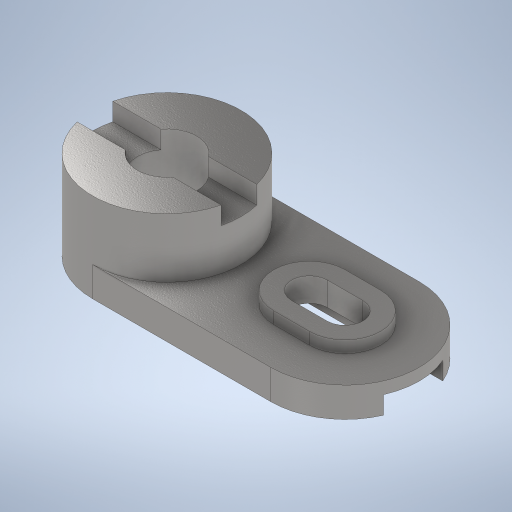
# Autodesk Inventor part: slider
Saved by Autodesk Inventor 2024 (Build 280153000, 153)
## iProperties
Created: 2024-02-08
Part Number: slider
Material: Stahl, galvanisiert
Document SubType Name: Modeling
Designer: ffogue
Density: 7.85 g/cm^3
Appearance: Galvanisiert
Author: ffogue
Autodesk Inventor part; units mm, degrees
ref_plane "XZ Plane" through (0, 0, 0) normal (0, 1, 0) x (-1, 0, 0)
ref_plane "XY Plane" through (0, 0, 0) normal (0, 0, 1) x (1, 0, 0)
sketch "Skizze1" plane through (0, 0, 0) normal (0, 0, 1) x (1, 0, 0)
  line L0 (0, 25) -> (60, 25)
  line L1 (0, -25) -> (60, -25)
  circle A0 centre (0, 0) radius 25
  arc A1 (60, -25) -> (60, 25) centre (60, 0) ccw
  line L2 (0, 0) -> (60, 0) construction
  point P0 (0, 0)
  dimension "d1" = 25
  dimension "d2" = 50
  dimension "d3" = 60
  constraints: 6 end point, 4 point on circle, 3 horizontal, 2 centre point, 2 tangent, 1 coincident, 1 vertical alignment
  measures "d1" radius of A1
  measures "d2" diameter of A0
  measures "d3" distance of L2.end point (0, 0)
extrude "Extrusion1" add sketch "Skizze1" along normal blind 10 contours L0 A1 L1 A0
extrude "Extrusion2" add sketch "Skizze1" along normal blind 30 contours A0
sketch "Skizze3" plane through (0, 0, 30) normal (0, 0, 1) x (1, 0, 0)
  circle A0 centre (0, 0) radius 25 projected
  line L0 (-24.2693, 6) -> (24.2693, 6)
  line L1 (-24.2693, -6) -> (24.2693, -6)
  line L2 (-25, 0) -> (25, 0) construction
  point P0 (0, 0)
  point P1 (0, 0)
  dimension "d11" = 12
  constraints: 6 end point, 6 point on circle, 2 horizontal, 1 coincident, 1 midpoint, 1 parallel, 1 other
  measures "d11" distance between parallel lines of L1 L0
extrude "Extrusion4" cut sketch "Skizze3" against normal blind 6 contours A0 L1 L0
sketch "Skizze4" plane through (0, 0, 30) normal (0, 0, 1) x (1, 0, 0)
  circle A0 centre (0, 0) radius 10
  dimension "d14" = 20
  constraints: 1 centre point, 1 coincident
  measures "d14" diameter of A0
extrude "Extrusion5" cut sketch "Skizze4" against normal up to surface (30 mm away)
sketch "Skizze5" plane through (0, 0, 10) normal (0, 0, 1) x (1, 0, 0)
  line L0 (48, 0) -> (60, 0) construction
  line L1 (48, -6) -> (60, -6)
  line L2 (60, 6) -> (48, 6)
  arc A0 (48, 6) -> (48, -6) centre (48, 0) ccw
  arc A1 (60, -6) -> (60, 6) centre (60, 0) ccw
  line L3 (48, 0) -> (60, 0) construction
  line L4 (48, -12) -> (60, -12)
  line L5 (60, 12) -> (48, 12)
  arc A2 (48, 12) -> (48, -12) centre (48, 0) ccw
  arc A3 (60, -12) -> (60, 12) centre (60, 0) ccw
  point P0 (0, 0)
  point P1 (54, 0)
  point P2 (54, 0)
  dimension "d17" = 12
  dimension "d18" = 60
  dimension "d19" = 6
  dimension "d20" = 12
  constraints: 16 end point, 8 point on circle, 8 tangent, 4 centre point, 3 equal length, 2 midpoint, 1 horizontal, 1 horizontal alignment
  measures "d17" distance of L0.end L0.start
  measures "d18" distance of point (0, 0) L0.end
  measures "d19" radius of A0
  measures "d20" radius of A2
extrude "Extrusion6" cut sketch "Skizze5" against normal up to surface (10 mm away) contours A0 L2 A1 L1
extrude "Extrusion7" add sketch "Skizze5" along normal blind 4
ref_plane "Arbeitsebene2" through (85, 0, 0) normal (1, 0, 0) x (0, 1, 0)
sketch "Skizze6" plane through (85, 0, 0) normal (1, 0, 0) x (0, 1, 0)
  line L0 (25, 0) -> (-25, 0) projected
  line L1 (-10, 0) -> (-10, 6)
  line L2 (-10, 6) -> (10, 6)
  line L3 (10, 6) -> (10, -0.2109)
  line L4 (0, 0) -> (0, 8.6058) construction
  line L5 (25, 10) -> (-25, 10) projected
  point P0 (0, 6)
  point P1 (0, 10)
  point P2 (10, 0)
  dimension "d26" = 20
  dimension "d27" = 4
  constraints: 8 end point, 2 midpoint, 1 horizontal, 1 perpendicular, 1 point on line, 1 vertical alignment, 1 other
  measures "d26" distance between parallel lines of L3 L1
  measures "d27" distance between parallel lines of L2 L5
extrude "Extrusion8" cut sketch "Skizze6" against normal through all
